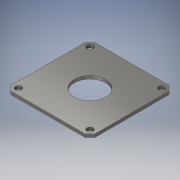
# Autodesk Inventor part: weldpart
Saved by Autodesk Inventor 2018 (Build 220112000, 112)
## iProperties
Created: 2019-03-04
Part Number: weldpart
Material: Stainless Steel
Document SubType Name: Modeling
Designer: freyja
Density: 8 g/cm^3
Appearance: Semi-Polished
Author: freyja
Autodesk Inventor part; units mm, degrees
ref_plane "YZ Plane" through (0, 0, 0) normal (1, 0, 0) x (0, 1, 0)
ref_plane "XZ Plane" through (0, 0, 0) normal (0, 1, 0) x (-1, 0, 0)
ref_plane "XY Plane" through (0, 0, 0) normal (0, 0, 1) x (1, 0, 0)
sketch "Sketch1" plane through (0, 0, 0) normal (0, 1, 0) x (-1, 0, 0)
  circle A0 centre (0, 0) radius 12.7
  line L0 (34.29, 34.29) -> (-34.29, 34.29)
  line L1 (-34.29, 34.29) -> (-34.29, -34.29)
  line L2 (-34.29, -34.29) -> (34.29, -34.29)
  line L3 (34.29, -34.29) -> (34.29, 34.29)
  line L4 (34.29, 34.29) -> (-34.29, -34.29) construction
  line L5 (-34.29, 34.29) -> (34.29, -34.29) construction
  dimension "d0" = 25.4
  dimension "d4" = 68.58
  dimension "d5" = 68.58
  constraints: 12 end point, 2 midpoint, 2 parallel, 1 centre point, 1 coincident, 1 horizontal, 1 perpendicular
  measures "d0" diameter of A0
  measures "d4" distance of L2.end L1.end
  measures "d5" distance between parallel lines of L0 L2
extrude "Extrusion1" add sketch "Sketch1" along normal blind 2.54
sketch "Sketch2" plane through (0, 2.54, 0) normal (0, 1, 0) x (1, 0, 0)
  line L0 (-29.21, -29.21) -> (29.21, -29.21) construction
  line L1 (29.21, -29.21) -> (29.21, 29.21) construction
  line L2 (29.21, 29.21) -> (-29.21, 29.21) construction
  line L3 (-29.21, 29.21) -> (-29.21, -29.21) construction
  line L4 (-29.21, -29.21) -> (29.21, 29.21) construction
  line L5 (29.21, -29.21) -> (-29.21, 29.21) construction
  line L6 (34.29, 34.29) -> (-34.29, 34.29) projected
  line L7 (34.29, -34.29) -> (34.29, 34.29) projected
  point P0 (0, 0)
  dimension "d15" = 5.08
  dimension "d16" = 5.08
  constraints: 12 end point, 4 coincident, 2 midpoint, 2 parallel, 1 horizontal, 1 perpendicular
  measures "d15" distance between parallel lines of L2 L6
  measures "d16" distance between parallel lines of L7 L1
hole "Hole1" at (-29.21, 2.54, -29.21) at (29.21, 2.54, -29.21) at (29.21, 2.54, 29.21) at (-29.21, 2.54, 29.21) direction (0, -1, 0) diameter 5.1054 end through all clearance for "Flat Head Machine Screw (82)" size "#10" standard "Ansi Unified Screw Threads"
sketch "Sketch3" plane through (0, 2.54, 0) normal (0, 1, 0) x (1, 0, 0)
  circle A0 centre (0, 0) radius 38.1
  circle A1 centre (0, 0) radius 12.7 projected
  circle A2 centre (0, 0) radius 25.4
  circle A3 centre (0, 0) radius 47.7012
  dimension "d17" = 76.2
  dimension "d18" = 50.8
  dimension "d19" = 95.4024
  constraints: 3 centre point, 3 coincident
  measures "d17" diameter of A0
  measures "d18" diameter of A2
  measures "d19" diameter of A3
sketch "Sketch4" plane through (0, 2.54, 0) normal (0, 1, 0) x (1, 0, 0)
  circle A0 centre (0, 0) radius 12.7 projected
  circle A1 centre (0, 0) radius 45.72
  dimension "d20" = 91.44
  constraints: 1 centre point, 1 coincident
  measures "d20" diameter of A1
extrude "Extrusion2" cut sketch "Sketch4" against normal blind 25.4 keep common part
body "Solid1"
